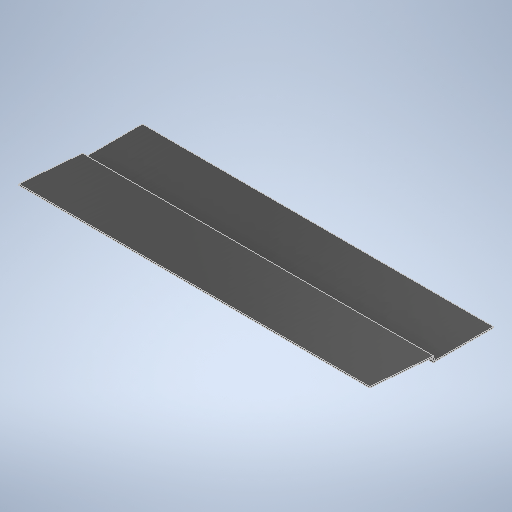
# Autodesk Inventor part: Second_Shingle_Over_Intake_Vent_With_Length_36.45_Inches
Saved by Autodesk Inventor 2025.1 (Build 291241020, 241B)
## iProperties
Created: 2024-10-02
Part Number: Second_Shingle_Over_Intake_Vent_With_Length_36.45_Inches
Material: Generic
Document SubType Name: Modeling
Designer: Tom
Density: 1 g/cm^3
Appearance: Dark Gray
Author: Tom
Autodesk Inventor part; units mm, degrees
ref_plane "YZ Plane" through (0, 0, 0) normal (1, 0, 0) x (0, 1, 0)
ref_plane "XZ Plane" through (0, 0, 0) normal (0, 1, 0) x (-1, 0, 0)
ref_plane "XY Plane" through (0, 0, 0) normal (0, 0, 1) x (1, 0, 0)
sketch "Sketch1" plane through (0, 0, 0) normal (1, 0, 0) x (0, 1, 0)
  line L0 (0, 0) -> (0, 597.7382)
  line L1 (0, 0) -> (3.175, 0)
  line L2 (3.175, 0) -> (3.175, 594.5632)
  line L3 (3.175, 594.5632) -> (9.906, 594.5632)
  line L4 (9.906, 594.5632) -> (15.756, 595.9828)
  line L5 (0, 597.7382) -> (9.5263, 597.7382)
  line L6 (9.5263, 597.7382) -> (12.7824, 598.5283)
  line L7 (41.2921, 902.0052) -> (15.756, 595.9828)
  line L8 (12.7824, 598.5283) -> (38.1281, 902.2692)
  line L9 (38.1281, 902.2692) -> (41.2921, 902.0052)
  line L10 (41.2921, 902.0052) -> (44.4671, 901.7403)
  line L11 (44.4671, 901.7403) -> (18.7409, 593.44)
  line L12 (18.7409, 593.44) -> (10.2857, 591.3882)
  line L13 (10.2857, 591.3882) -> (6.35, 591.3882)
  line L14 (6.35, 591.3882) -> (6.35, 574.5988)
  line L15 (6.35, 574.5988) -> (3.175, 574.5988)
  line L16 (44.4671, 901.7403) -> (47.6311, 901.4763)
  line L17 (47.6311, 901.4763) -> (21.7146, 590.8944)
  line L18 (21.7146, 590.8944) -> (10.6654, 588.2132)
  line L19 (10.6654, 588.2132) -> (9.525, 588.2132)
  line L20 (9.525, 588.2132) -> (9.525, 432.9684)
  line L21 (9.525, 432.9684) -> (6.35, 432.9684)
  line L22 (6.35, 432.9684) -> (6.35, 574.5988)
  line L23 (32.5862, 759.3601) -> (35.7502, 759.0961)
  point P0 (14.5133, 592.4141)
  dimension "d0" = 594.5632
  dimension "d1" = 3.175
  dimension "d2" = 6.731
  dimension "d7" = 3.175
  dimension "d8" = 6.0198
  dimension "d9" = 166.36
  dimension "d10" = 3.175
  dimension "d11" = 108.41
  dimension "d12" = 3.175
  dimension "d13" = 307.086
  dimension "d18" = 3.175
  dimension "d20" = 307.1025
  dimension "d21" = 8.7006
  dimension "d22" = 3.175
  dimension "d23" = 3.175
  dimension "d24" = 3.9357
  dimension "d25" = 16.7894
  dimension "d28" = 3.175
  dimension "d29" = 3.186
  dimension "d30" = 3.175
  dimension "d32" = 3.175
  dimension "d33" = 3.175
  dimension "d34" = 142.875
  dimension "d35" = 168.7862
  dimension "d36" = 11.3698
  dimension "d37" = 1.1404
  dimension "d38" = 155.2448
  constraints: 48 end point, 11 perpendicular, 6 parallel, 3 horizontal, 3 point on line, 1 collinear, 1 midpoint, 1 vertical
  measures "d0" distance of L1.end L2.end
  measures "d1" distance between parallel lines of L2 L0
  measures "d2" distance of L2.end L3.end
  measures "d7" distance between parallel lines of L5 L3
  measures "d8" distance of L3.end L4.end
  measures "d9" angle of L3 L4
  measures "d10" distance between parallel lines of L6 L4
  measures "d11" angle of L4 L7
  measures "d12" distance between parallel lines of L7 L8
  measures "d13" distance of L7.start L4.end
  measures "d18" distance between parallel lines of L12 L4
  measures "d20" distance of L4.end L10.end
  measures "d21" distance of L11.end L12.end
  measures "d22" distance between parallel lines of L13 L3
  measures "d23" distance between parallel lines of L2 L14
  measures "d24" distance of L12.end L13.end
  measures "d25" distance of L13.end L14.end
  measures "d28" distance between parallel lines of L17 L11
  measures "d29" distance between parallel lines of L11 L7
  measures "d30" distance from line of L18 point (14.513, 592.414)
  measures "d32" distance between parallel lines of L20 L22
  measures "d33" distance between parallel lines of L19 L13
  measures "d34" distance between parallel lines of L16 L23
  measures "d35" distance of L17.end L23.end
  measures "d36" distance of L17.end L18.end
  measures "d37" distance of L18.end L19.end
  measures "d38" distance of L19.end L20.end
extrude "Extrusion3" add sketch "Sketch1" along normal blind 925.83 contours L14 L13 L12 L11 L23 L17 L18 L19 L20 L21 L22
body "Solid3"
